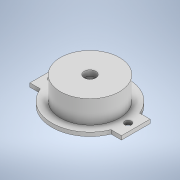
# Autodesk Inventor part: magnetholder
Saved by Autodesk Inventor 2021.5 (Build 255421000, 421)
## iProperties
Created: 2024-11-28
Part Number: magnetholder
Material: Generic
Document SubType Name: Modeling
Designer: email
Density: 1 g/cm^3
Appearance: Default
Author: email
Autodesk Inventor part; units mm, degrees
ref_plane "YZ Plane" through (0, 0, 0) normal (1, 0, 0) x (0, 1, 0)
ref_plane "XZ Plane" through (0, 0, 0) normal (0, 1, 0) x (-1, 0, 0)
ref_plane "XY Plane" through (0, 0, 0) normal (0, 0, 1) x (1, 0, 0)
sketch "Sketch1" plane through (0, 0, 0) normal (0, 1, 0) x (-1, 0, 0)
  circle A0 centre (0, 0) radius 1.5
  circle A1 centre (0, 0) radius 20
  line L0 (24, -7.5) -> (-24, -7.5)
  line L1 (-24, -7.5) -> (-24, 7.5)
  line L2 (-24, 7.5) -> (24, 7.5)
  line L3 (24, 7.5) -> (24, -7.5)
  line L4 (24, -7.5) -> (-24, 7.5) construction
  line L5 (-24, -7.5) -> (24, 7.5) construction
  circle A2 centre (0, 0) radius 11
  circle A3 centre (20, 0) radius 1.75
  circle A4 centre (-20, 0) radius 1.75
  circle A5 centre (0, 0) radius 15.5
  point P0 (-18.5405, -7.5)
  point P1 (18.5405, -7.5)
  point P2 (18.5405, 7.5)
  point P3 (-18.5405, 7.5)
  dimension "d0" = 40
  dimension "d1" = 48
  dimension "d2" = 15
  dimension "d3" = 22
  dimension "d4" = 3.5
  dimension "d5" = 3.5
  dimension "d6" = 31
  constraints: 12 end point, 6 centre point, 3 coincident, 2 midpoint, 2 parallel, 2 point on circle, 1 horizontal, 1 perpendicular
  measures "d0" diameter of A1
  measures "d1" distance of L0.start L0.end
  measures "d2" distance of L0.end L1.end
  measures "d3" diameter of A2
  measures "d4" diameter of A3
  measures "d5" diameter of A4
  measures "d6" diameter of A5
extrude "Extrusion1" add sketch "Sketch1" along normal blind 2 contours A3 A1 L0 A5 L2 | A1 L2 L3 L0 A3 | L2 A5 A1 | A1 L0 A5 | L2 A5 L0 A1 A4 | A1 A4 L0 L1 L2
extrude "Extrusion2" add sketch "Sketch1" along normal blind 9 contours A5 L0 A2 L2 | L2 A2 A5 | A5 L0 A2 | L2 A2 L0 A5
sketch "Sketch2" plane through (0, 9, 0) normal (0, 1, 0) x (1, 0, 0)
  circle A0 centre (0, 0) radius 15.5
  circle A1 centre (0, 0) radius 8.3846
  circle A2 centre (0, 0) radius 3.075
  dimension "d11" = 31
  dimension "d12" = 6.15
  constraints: 3 centre point, 3 coincident
  measures "d11" diameter of A0
  measures "d12" diameter of A2
extrude "Extrusion3" add sketch "Sketch2" along normal blind 5 contours A0 | A1
extrude "Extrusion4" add sketch "Sketch2" along normal blind 2 contours A1 | A2
body "Solid1"
